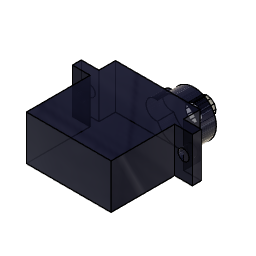
Servo (Autodesk Fusion 360 design; units mm, degrees)
Autodesk Fusion 360 part; units mm, degrees
sketch "Sketch1" plane through (0, 0, 0) normal (0, 0, 1) x (1, 0, 0)
  line L0 (11.5, -12.1) -> (-11.5, -12.1)
  line L1 (-11.5, 12.1) -> (11.5, 12.1)
  line L2 (11.5, -12.1) -> (-11.5, 12.1) construction
  line L3 (-11.5, -12.1) -> (11.5, 12.1) construction
  line L4 (11.5, 7.6) -> (16.3, 7.6)
  line L5 (16.3, 7.6) -> (16.3, 5.2)
  line L6 (16.3, 5.2) -> (11.5, 5.2)
  line L7 (-16.3, 5.2) -> (-11.5, 5.2)
  line L8 (-16.3, 7.6) -> (-16.3, 5.2)
  line L9 (-11.5, 7.6) -> (-16.3, 7.6)
  line L10 (11.5, 12.1) -> (11.5, 7.6)
  line L11 (11.5, 5.2) -> (11.5, -12.1)
  line L12 (-11.5, -12.1) -> (-11.5, 5.2)
  line L13 (-11.5, 7.6) -> (-11.5, 12.1)
  dimension "d1" = 23
  dimension "d2" = 24.2
  dimension "d3" = 4.5
  dimension "d4" = 4.8
  dimension "d5" = 2.4
  constraint horizontal L0
  constraint perpendicular L0 L12
  constraint parallel L0 L1
  constraint parallel L10 L12
  constraint coincident L2 origin
  constraint coincident L3 origin
  constraint horizontal L4
  constraint vertical L5
  constraint horizontal L6
  constraint collinear L10 L11
  constraint collinear L12 L13
  measures "d1" distance of L1.start L1.end
  measures "d2" distance of L0.end L1.start
  measures "d3" distance of L1.end L4.start
  measures "d4" distance of L4.start L4.end
  measures "d5" distance of L4.start L6.end
extrude "Extrude1" add sketch "Sketch1" along normal blind 12.1
sketch "Sketch2" plane through (0, 7.6, 0) normal (0, 1, 0) x (-1, 0, 0)
  line L0 (-16.3, 0) -> (-11.5, 0)
  line L1 (-11.5, 0) -> (-11.5, 12.1)
  line L2 (-11.5, 12.1) -> (-16.3, 12.1)
  line L3 (-16.3, 12.1) -> (-16.3, 0)
  circle A0 centre (14, 6) radius 1.5
  circle A1 centre (-13.9, 6.05) radius 1.5
  dimension "d8" = 3
  dimension "d9" = 3
  measures "d8" diameter of A0
  measures "d9" diameter of A1
extrude "Extrude2" cut sketch "Sketch2" against normal blind 5 contours A0 | A1
sketch "Sketch3" plane through (0, 12.1, 0) normal (0, 1, 0) x (-1, 0, 0)
  line L0 (-11.5, 0) -> (11.5, 0)
  line L1 (11.5, 0) -> (11.5, 12.1)
  line L2 (11.5, 12.1) -> (-11.5, 12.1)
  line L3 (-11.5, 12.1) -> (-11.5, 0)
  line L4 (0.6, 6.05) -> (0.65, 6.05)
  arc A0 (0.0672, 3.5675) -> (0.0672, 8.5325) centre (0.65, 6.05) ccw
  arc A1 (0.0672, 8.5325) -> (0.0672, 3.5675) centre (-5.45, 6.05) ccw
  dimension "d12" = 6.1
  dimension "d13" = 5.1
  constraint tangent L3 A1
  constraint tangent L2 A1
  constraint tangent L0 A1
  constraint horizontal L4
  constraint coincident L4.end A0.centre
  measures "d12" distance of A1.centre L4.end
  measures "d13" diameter of A0
extrude "Extrude3" add sketch "Sketch3" along normal blind 4.4 contours A0 A1
sketch "Sketch4" plane through (0, 16.5, 0) normal (0, 1, 0) x (-1, 0, 0)
  arc A0 (0.0672, 8.5325) -> (0.0672, 3.5675) centre (-5.45, 6.05) ccw
  arc A1 (0.0672, 3.5675) -> (0.0672, 8.5325) centre (0.65, 6.05) ccw
  circle A2 centre (-5.45, 6.05) radius 2.35
  line L0 (-4.4572, 3.92) -> (-3.5252, 4.7018)
  line L1 (-3.5252, 4.7018) -> (-3.109, 5.8448)
  line L2 (-3.109, 5.8448) -> (-3.32, 7.0428)
  line L3 (-3.32, 7.0428) -> (-4.1018, 7.9748)
  line L4 (-4.1018, 7.9748) -> (-5.2448, 8.391)
  line L5 (-5.2448, 8.391) -> (-6.4428, 8.18)
  line L6 (-6.4428, 8.18) -> (-7.3748, 7.3982)
  line L7 (-7.3748, 7.3982) -> (-7.791, 6.2552)
  line L8 (-7.791, 6.2552) -> (-7.58, 5.0572)
  line L9 (-7.58, 5.0572) -> (-6.7982, 4.1252)
  line L10 (-6.7982, 4.1252) -> (-5.6552, 3.709)
  line L11 (-5.6552, 3.709) -> (-4.4572, 3.92)
  point P0 (-5.45, 6.05)
  dimension "d16" = 4.7
  constraint concentric A0 A2
  constraint coincident A2 L0.start
  constraint coincident P0 A0.centre
  measures "d16" diameter of A2
extrude "Extrude4" add sketch "Sketch4" along normal blind 3.6 contours L0 L1 L2 L3 L4 L5 L6 L7 L8 L9 L10 L11
